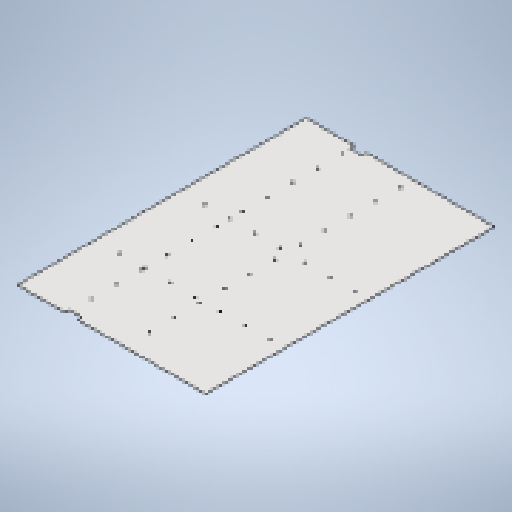
# Autodesk Inventor part: GnG frame 2 floor sheet 8
Saved by Autodesk Inventor 2025 (Build 290162010, 162A)
## iProperties
Created: 2025-10-28
Part Number: GnG frame 2 floor sheet 8
Material: Stainless Steel
Document SubType Name: Sheet Metal
Designer: admin
Mass: 280.619 g
Surface Area: 364.406 cm^2
Volume: 35.0774 cm^3
Density: 8 g/cm^3
Sheet Metal Rule: AISI304 3mm Die 32
Sheet Metal Width: 1500,000 mm
Sheet Metal Length: 2300,000 mm
Sheet Metal Area: 3450000,000 mm^2
Appearance: Default
Flat Pattern Width: 150 cm
Flat Pattern Length: 230 cm
Flat Pattern Area: 34500 cm^2
Author: admin
Autodesk Inventor part; units mm, degrees
ref_plane "YZ Plane" through (0, 0, 0) normal (1, 0, 0) x (0, 1, 0)
ref_plane "XZ Plane" through (0, 0, 0) normal (0, 1, 0) x (-1, 0, 0)
ref_plane "XY Plane" through (0, 0, 0) normal (0, 0, 1) x (1, 0, 0)
sketch "Sketch1" plane through (0, 0, 0) normal (0, 0, 1) x (1, 0, 0)
  line L0 (0, 0) -> (-1500, 0)
  line L1 (-1500, 0) -> (-1500, -2300)
  line L2 (-1500, -2300) -> (0, -2300)
  line L3 (0, -2300) -> (0, 0)
  line L4 (0, 0) -> (-65, 0)
  line L5 (-65, 0) -> (-65, -35)
  line L6 (-65, -35) -> (0, -35)
  line L7 (0, -35) -> (0, 0)
  line L8 (0, -2300) -> (-65, -2300)
  line L9 (-65, -2300) -> (-65, -2265)
  line L10 (-65, -2265) -> (0, -2265)
  line L11 (0, -2265) -> (0, -2300)
  line L12 (-1500, 0) -> (-1435, 0)
  line L13 (-1435, 0) -> (-1435, -35)
  line L14 (-1435, -35) -> (-1500, -35)
  line L15 (-1500, -35) -> (-1500, 0)
  line L16 (-1500, -2300) -> (-1435, -2300)
  line L17 (-1435, -2300) -> (-1435, -2265)
  line L18 (-1435, -2265) -> (-1500, -2265)
  line L19 (-1500, -2265) -> (-1500, -2300)
  line L20 (-1120, -2300) -> (-1020, -2300)
  line L21 (-1020, -2300) -> (-1020, -2265)
  line L22 (-1020, -2265) -> (-1120, -2265)
  line L23 (-1120, -2265) -> (-1120, -2300)
  line L24 (-1120, 0) -> (-1020, 0)
  line L25 (-1020, 0) -> (-1020, -35)
  line L26 (-1020, -35) -> (-1120, -35)
  line L27 (-1120, -35) -> (-1120, 0)
  point P0 (0, -35)
  point P1 (-65, 0)
  point P2 (0, -2265)
  point P3 (-1020, -2300)
  point P4 (-1020, 0)
  point P5 (-1435, 0)
  dimension "d22" = 1500
  dimension "d23" = 2300
  dimension "d24" = 65
  dimension "d25" = 35
  dimension "d28" = 100
  dimension "d29" = 955
  measures "d22" distance of L2.end L1.end
  measures "d23" distance of L1.end L0.end
  measures "d24" distance of L6.end L5.end
  measures "d25" distance of L5.end L4.end
  measures "d28" distance of L25.end L26.end
  measures "d29" distance between parallel lines of L5 L25
extrude "Plate1" add sketch "Sketch1" along normal blind 3 contours L3 L6 L5 L0 | L5 L6 L3 L10 L9 L2 L21 L22 L23 L17 L18 L1 L14 L13 L0 L27 L26 L25 | L3 L2 L9 L10 | L13 L14 L1 L0 | L18 L17 L2 L1
sketch "Sketch5" plane through (0, 0, 3) normal (0, 0, 1) x (1, 0, 0)
  line L0 (0, 0) -> (-100, 0) construction
  line L1 (-100, 0) -> (-100, -2) construction
  line L2 (-100, -2) -> (0, -2) construction
  line L3 (0, -2) -> (0, 0) construction
  line L4 (-100, 0) -> (-101.5248, -4.6556)
  arc A0 (-102.4752, -4.6556) -> (-101.5248, -4.6556) centre (-102, -4.5) ccw
  line L5 (-102.4752, -4.6556) -> (-104, 0)
  line L6 (-104, 0) -> (-100, 0)
  line L7 (-104, 0) -> (-106, 0) construction
  line L8 (-106, 0) -> (-108, 0)
  line L9 (-108, 0) -> (-108, -5)
  line L10 (-108, -5) -> (-106, -5)
  line L11 (-106, -5) -> (-106, 0)
  line L12 (-108, 0) -> (-110, 0) construction
  line L13 (-110, 0) -> (-112, 0)
  line L14 (-112, 0) -> (-112, -5)
  line L15 (-112, -5) -> (-110, -5)
  line L16 (-110, -5) -> (-110, 0)
  line L17 (-112, 0) -> (-114, 0) construction
  line L18 (-114, 0) -> (-116, 0)
  line L19 (-116, 0) -> (-116, -5)
  line L20 (-116, -5) -> (-114, -5)
  line L21 (-114, -5) -> (-114, 0)
  line L22 (-116, 0) -> (-118, 0) construction
  line L23 (-118, 0) -> (-120, 0)
  line L24 (-120, 0) -> (-120, -5)
  line L25 (-120, -5) -> (-118, -5)
  line L26 (-118, -5) -> (-118, 0)
  line L27 (-120, 0) -> (-125, 0) construction
  line L28 (-125, 0) -> (-130, 0) construction
  circle A1 centre (-125, 0) radius 1
  circle A2 centre (-130, 0) radius 1
  point P0 (0, 0)
  point P1 (-102, 0)
  dimension "d30" = 100
  dimension "d31" = 2
  dimension "d32" = 5
  dimension "d33" = 4
  dimension "d34" = 0.5
  dimension "d35" = 5
  dimension "d36" = 5
  dimension "d37" = 5
  dimension "d38" = 2
  constraints: 58 end point, 11 horizontal, 10 equal length, 10 parallel, 5 perpendicular, 4 coincident, 3 centre point, 3 tangent, 2 point on circle, 1 equal radius, 1 midpoint, 1 point on line, 1 vertical alignment
  measures "d30" distance of L2.end L1.end
  measures "d31" distance of L1.end L0.end
  measures "d32" distance of L9.end L9.start
  measures "d33" distance of L5.end L0.end
  measures "d34" radius of A0
  measures "d35" distance of L15.start L13.end
  measures "d36" distance of L19.end L19.start
  measures "d37" distance of L24.end L24.start
  measures "d38" diameter of A1
extrude "Cut1" cut sketch "Sketch5" against normal blind 3 contours L4 A0 L5 L6 | A1 | A2
sketch "Sketch6" plane through (0, 0, 3) normal (0, 0, 1) x (1, 0, 0)
  line L0 (-102.4752, -4.6556) -> (-104, 0) construction
  line L1 (-124, 0) -> (-104, 0) construction
  arc A0 (-126, 0) -> (-124, 0) centre (-125, 0) ccw construction
  line L2 (-129, 0) -> (-126, 0) construction
  arc A1 (-131, 0) -> (-129, 0) centre (-130, 0) ccw construction
  line L3 (-1020, 0) -> (-131, 0) construction
  line L4 (-1020, -35) -> (-1020, 0) construction
  line L5 (-1120, -35) -> (-1020, -35) construction
  line L6 (-1120, 0) -> (-1120, -35) construction
  line L7 (-1500, 0) -> (-1120, 0) construction
  line L8 (-1500, -2300) -> (-1500, 0) construction
  line L9 (-1120, -2300) -> (-1500, -2300) construction
  line L10 (-1120, -2265) -> (-1120, -2300) construction
  line L11 (-1020, -2265) -> (-1120, -2265) construction
  line L12 (-1020, -2300) -> (-1020, -2265) construction
  line L13 (0, -2300) -> (-1020, -2300) construction
  line L14 (0, 0) -> (0, -2300) construction
  line L15 (-100, 0) -> (0, 0) construction
  line L16 (-100, 0) -> (-101.5248, -4.6556) construction
  arc A2 (-102.4752, -4.6556) -> (-101.5248, -4.6556) centre (-102, -4.5) ccw construction
  line L17 (0, -2300) -> (0, 0) construction
  line L18 (0, -1000) -> (-1500, -1000) construction
  line L19 (-1500, -1675) -> (0, -1675) construction
  line L20 (-650, 0) -> (-650, -2300) construction
  line L21 (-1110, -2300) -> (-1110, 0) construction
  circle A3 centre (-650, -2100) radius 7.5
  circle A4 centre (-1110, -2100) radius 7.5
  circle A5 centre (-1310, -1675) radius 7.5
  circle A6 centre (-1310, -1000) radius 7.5
  circle A7 centre (-650, -1900) radius 7.5
  circle A8 centre (-1110, -1900) radius 7.5
  circle A9 centre (-650, -1700) radius 7.5
  circle A10 centre (-1110, -1700) radius 7.5
  circle A11 centre (-650, -1500) radius 7.5
  circle A12 centre (-1110, -1500) radius 7.5
  circle A13 centre (-650, -1300) radius 7.5
  circle A14 centre (-1110, -1300) radius 7.5
  circle A15 centre (-650, -1100) radius 7.5
  circle A16 centre (-1110, -1100) radius 7.5
  circle A17 centre (-650, -900) radius 7.5
  circle A18 centre (-1110, -900) radius 7.5
  circle A19 centre (-650, -700) radius 7.5
  circle A20 centre (-1110, -700) radius 7.5
  circle A21 centre (-650, -500) radius 7.5
  circle A22 centre (-1110, -500) radius 7.5
  circle A23 centre (-650, -300) radius 7.5
  circle A24 centre (-1110, -300) radius 7.5
  circle A25 centre (-650, -100) radius 7.5
  circle A26 centre (-1110, -100) radius 7.5
  circle A27 centre (-1110, -1675) radius 7.5
  circle A28 centre (-1110, -1000) radius 7.5
  circle A29 centre (-910, -1675) radius 7.5
  circle A30 centre (-910, -1000) radius 7.5
  circle A31 centre (-710, -1675) radius 7.5
  circle A32 centre (-710, -1000) radius 7.5
  circle A33 centre (-510, -1675) radius 7.5
  circle A34 centre (-510, -1000) radius 7.5
  circle A35 centre (-310, -1675) radius 7.5
  circle A36 centre (-310, -1000) radius 7.5
  circle A37 centre (-110, -1675) radius 7.5
  circle A38 centre (-110, -1000) radius 7.5
  dimension "d41" = 390
  dimension "d42" = 850
  dimension "d43" = 1300
  dimension "d44" = 625
  dimension "d45" = 15
  dimension "d46" = 200
  dimension "d47" = 190
  dimension "d50" = 200
  dimension "d57" = 200
  constraints: 36 centre point, 12 point on line, 8 end point, 4 perpendicular, 3 equal radius, 1 horizontal, 1 horizontal alignment, 1 vertical, 1 vertical alignment, 64 other
  measures "d41" distance between parallel lines of L8 L21
  measures "d42" distance between parallel lines of L8 L20
  measures "d43" distance between parallel lines of L9 L18
  measures "d44" distance between parallel lines of L9 L19
  measures "d45" diameter of A3
  measures "d46" distance from line of L9 A3.centre
  measures "d47" distance from line of L8 A6.centre
  measures "d50" distance of A3.centre A7.centre
  measures "d57" distance of A5.centre A27.centre
extrude "Cut2" cut sketch "Sketch6" against normal blind 3
equation "\"d33\" = 2 * d31"
equation "\"d34\" = 0.25 * d31"
equation "\"d38\" = d31"
equation "\"d39\" = Thickness"
equation "\"d50\" = d46"
equation "\"d57\" = d46"
equation "\"d62\" = Thickness"
equation "\"d2\" = Thickness"
equation "\"BendReliefWidth\" = Thickness"
equation "\"BendReliefDepth\" = 0.5 * Thickness"
equation "\"CornerReliefSize\" = 4 * Thickness"
equation "\"MinimumRemnant\" = 2 * Thickness"
equation "\"TransitionRadius\" = BendRadius"
equation "\"JacobiRadiusSize\" = BendRadius"
equation "\"GapSize\" = Thickness"
equation "\"Thickness\" = 3"
equation "\"BendRadius\" = 5"
body "Solid1"
